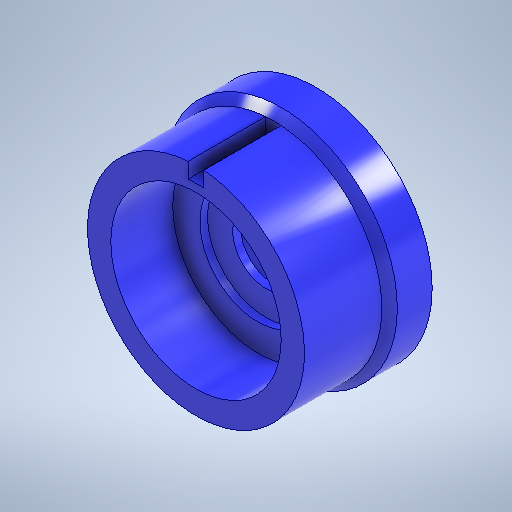
# Autodesk Inventor part: bielle côté 2
Saved by Autodesk Inventor 2026.2 (Build 302298010, 298A)
## iProperties
Created: 2026-03-16
Part Number: bielle côté 2
Material: Générique
Document SubType Name: Modeling
Designer: genon
Density: 1 g/cm^3
Appearance: Bleu - Peinture murale - Brillant
Author: genon
Autodesk Inventor part; units mm, degrees
ref_plane "YZ Plane" through (0, 0, 0) normal (1, 0, 0) x (0, 1, 0)
ref_plane "XZ Plane" through (0, 0, 0) normal (0, 1, 0) x (-1, 0, 0)
sketch "Esquisse1" plane through (0, 0, 0) normal (0, 0, 1) x (1, 0, 0)
  circle A0 centre (0, 0) radius 15
  line L0 (0, 0) -> (-10, 0)
  line L1 (0, 0) -> (0, 10)
  line L2 (0, 0) -> (10, 0)
  line L3 (0, 0) -> (0, -10)
  line L4 (0, -10) -> (10, 0)
  line L5 (10, 0) -> (0, 10)
  line L6 (0, 10) -> (-10, 0)
  line L7 (-10, 0) -> (0, -10)
  dimension "d0" = 30
  dimension "d1" = 10
  dimension "d2" = 10
  dimension "d3" = 10
  dimension "d4" = 10
  constraints: 16 end point, 2 horizontal, 2 vertical, 1 centre point, 1 coincident
  measures "d0" diameter of A0
  measures "d1" distance of L0.start L0.end
  measures "d2" distance of L0.start L1.end
  measures "d3" distance of L0.start L2.end
  measures "d4" distance of L0.start L3.end
extrude "Extrusion1" add sketch "Esquisse1" along normal blind 5.5
chamfer "Chanfrein1" distance 1 angle 45 1 edges at (-15, 0, 5.5)
sketch "Esquisse2" plane through (0, 0, 5.5) normal (0, 0, 1) x (1, 0, 0)
  circle A0 centre (0, 0) radius 11.5
  circle A1 centre (0, 0) radius 14
  line L0 (0, -10) -> (-10, 0) projected
  line L1 (0, 10) -> (10, 0) projected
  line L2 (-10, 0) -> (0, 10)
  line L3 (0, 10) -> (10, 0)
  line L4 (10, 0) -> (0, -10)
  line L5 (0, -10) -> (-10, 0)
  dimension "d10" = 23
  dimension "d26" = 28
  constraints: 8 end point, 3 perpendicular, 2 centre point, 2 coincident, 1 collinear
  measures "d10" diameter of A0
  measures "d26" diameter of A1
extrude "Extrusion2" add sketch "Esquisse2" along normal blind 1 contours A0 | A1 | L0 L2 L1 L4
sketch "Esquisse3" plane through (0, 0, 6.5) normal (0, 0, 1) x (1, 0, 0)
  circle A0 centre (0, 0) radius 11
  circle A1 centre (0, 0) radius 14
  dimension "d13" = 22
  dimension "d27" = 28
  constraints: 2 centre point, 2 coincident
  measures "d13" diameter of A0
  measures "d27" diameter of A1
extrude "Extrusion3" add sketch "Esquisse3" along normal blind 9
sketch "Esquisse4" plane through (0, 0, 6.5) normal (0, 0, 1) x (1, 0, 0)
  circle A0 centre (0, 0) radius 4.25
  dimension "d16" = 8.5
  constraints: 1 centre point, 1 coincident
  measures "d16" diameter of A0
extrude "Extrusion4" cut sketch "Esquisse4" against normal through all
ref_plane "Plan de construction1" through (0, 0, 15.5) normal (0, 0, -1) x (-1, 0, 0)
sketch "Esquisse6" plane through (0, 0, 15.5) normal (0, 0, -1) x (-1, 0, 0)
  circle A0 centre (0, 0) radius 14
  line L0 (0, 0) -> (0, 12)
  line L1 (0, 12) -> (-1, 12)
  line L2 (-1, 12) -> (-1, 13.9642)
  circle A1 centre (0, 0) radius 14 projected
  line L3 (0, 12) -> (1, 12)
  line L4 (1, 12) -> (1, 13.9642)
  dimension "d29" = 12
  dimension "d30" = 1
  dimension "d31" = 1
  constraints: 10 end point, 3 perpendicular, 2 point on circle, 1 centre point, 1 coincident, 1 point on line, 1 vertical
  measures "d29" distance of L0.start L0.end
  measures "d30" distance of L0.end L1.end
  measures "d31" distance of L0.end L3.end
extrude "Extrusion6" cut sketch "Esquisse6" along normal blind 10 contours L4 L3 L1 L2 A0 picked at (-0.4445, 12.6653)
sketch "Esquisse7" plane through (0, 0, 6.5) normal (0, 0, 1) x (1, 0, 0)
  circle A0 centre (0, 0) radius 11 projected
  circle A1 centre (0, 0) radius 7.5
  dimension "d34" = 15
  constraints: 1 centre point, 1 coincident
  measures "d34" diameter of A1
extrude "Extrusion7" add sketch "Esquisse7" along normal blind 1
